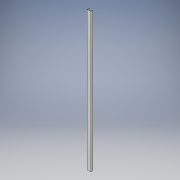
# Autodesk Inventor part: Grundstange Bauhaus_neu
Saved by Autodesk Inventor 2018.3 (Build 223284000, 284)
## iProperties
Created: 2019-01-17
Part Number: Grundstange Bauhaus_neu
Material: Generisch
Document SubType Name: Modeling
Designer: pgmadmin
Density: 1 g/cm^3
Appearance: Vorgabe
Author: pgmadmin
Autodesk Inventor part; units mm, degrees
ref_plane "YZ Plane" through (0, 0, 0) normal (1, 0, 0) x (0, 1, 0)
ref_plane "XZ Plane" through (0, 0, 0) normal (0, 1, 0) x (-1, 0, 0)
ref_plane "XY Plane" through (0, 0, 0) normal (0, 0, 1) x (1, 0, 0)
sketch "Skizze1" plane through (0, 0, 0) normal (0, 0, 1) x (1, 0, 0)
  line L0 (-10.9286, -11.051) -> (-10.9286, 3.949)
  line L1 (-10.9286, 3.949) -> (-9.4286, 3.949)
  line L2 (-9.4286, 3.949) -> (-9.4286, -9.551)
  line L3 (-9.4286, -9.551) -> (15.0714, -9.551)
  line L4 (15.0714, -9.551) -> (15.0714, 3.949)
  line L5 (15.0714, 3.949) -> (16.5714, 3.949)
  line L6 (16.5714, 3.949) -> (16.5714, -11.051)
  line L7 (16.5714, -11.051) -> (-10.9286, -11.051)
  point P0 (0, 0)
  dimension "d0" = 1.5
  dimension "d1" = 27.5
  dimension "d2" = 1.5
  dimension "d3" = 1.5
  dimension "d4" = 15
  dimension "d5" = 15
  constraints: 16 end point, 6 perpendicular, 2 vertical
  measures "d0" distance between parallel lines of L2 L0
  measures "d1" distance between parallel lines of L6 L0
  measures "d2" distance between parallel lines of L6 L4
  measures "d3" distance between parallel lines of L3 L7
  measures "d4" distance between parallel lines of L7 L1
  measures "d5" distance between parallel lines of L7 L5
extrude "Extrusion1" add sketch "Skizze1" along normal blind 1000
